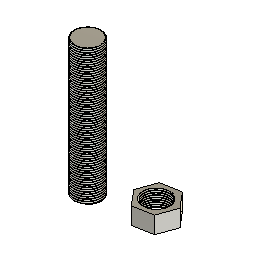
screw (Autodesk Fusion 360 design; units mm, degrees)
part number: 2025-09-17-23-51-49-752
Autodesk Fusion 360 part; units mm, degrees
sketch "Sketch1" plane through (0, 0, 0) normal (0, 0, 1) x (1, 0, 0)
  circle A0 centre (0, 0) radius 20
  dimension "d1" = 40
  constraint coincident A0.centre origin
  measures "d1" diameter of A0
extrude "Extrude1" add sketch "Sketch1" along normal blind 200 makes body 1
thread "Thread1" "ISO Metric profile 40.0 M40x3 M40x3 6g" major diameter 39.7645 minor diameter 36.3299 pitch 3 angle 60 modelled right hand crest width 0.4255 on face at (19.9006, -1.9914, 66.6667) crest through (19.8822, 0, -0.75) on bodies 1
sketch "Sketch2" plane through (0, 0, 0) normal (0, 0, 1) x (1, 0, 0)
  circle A0 centre (81.826, 19.6989) radius 20
  line L0 (91.7733, 47.2622) -> (62.9291, 42.0952)
  line L1 (62.9291, 42.0952) -> (52.9818, 14.5318)
  line L2 (52.9818, 14.5318) -> (71.8787, -7.8645)
  line L3 (71.8787, -7.8645) -> (100.7229, -2.6975)
  line L4 (100.7229, -2.6975) -> (110.6702, 24.8659)
  line L5 (110.6702, 24.8659) -> (91.7733, 47.2622)
  point P0 (81.826, 19.6989)
  dimension "d6" = 40
  constraint coincident P0 A0.centre
  measures "d6" diameter of A0
extrude "Extrude2" add sketch "Sketch2" along normal blind 25 separate body makes body 2
thread "Thread2" "ISO Metric profile 40.0 M40x3 M40x3 6H" major diameter 40.349 minor diameter 37.0024 pitch 3 angle 60 modelled right hand crest width 0.8179 on face at (101.7266, 17.7075, 8.3333) crest through (100.3272, 19.6989, 0.75) on bodies 2
